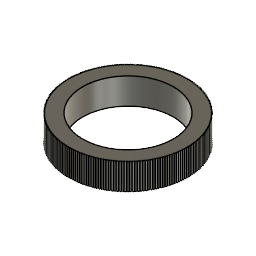
tyre (Autodesk Fusion 360 design; units mm, degrees)
Autodesk Fusion 360 part; units mm, degrees
note: some values were not read from the file. Set by a fixed rule: which sketch regions a step uses.
sketch "Sketch1" plane through (0, 0, 0) normal (0, 0, 1) x (1, 0, 0)
  circle A0 centre (0, 0) radius 17.25
  circle A1 centre (0, 0) radius 22.5
  dimension "d1" = 34.5
  dimension "d2" = 45
  constraint coincident A0.centre A1.centre
  constraint concentric A0 A1
  measures "d1" diameter of A0
  measures "d2" diameter of A1
extrude "Extrude1" add sketch "Sketch1" along normal blind 8
extrude "Extrude2" add 1 faces at (20.602, -1.9748, 8) along direction (0, 0, 1) blind 2
sketch "Sketch2" plane through (0, 0, 10) normal (0, 0, 1) x (-1, 0, 0)
  circle A0 centre (0, 0) radius 17.25
  circle A1 centre (0, 0) radius 22.5
  circle A2 centre (0, -22.5) radius 0.25
  circle A3 centre (0.7067, -22.4889) radius 0.25
  circle A4 centre (1.4128, -22.4556) radius 0.25
  circle A5 centre (2.1174, -22.4001) radius 0.25
  circle A6 centre (2.82, -22.3226) radius 0.25
  circle A7 centre (3.5198, -22.223) radius 0.25
  circle A8 centre (4.2161, -22.1015) radius 0.25
  circle A9 centre (4.9082, -21.9581) radius 0.25
  circle A10 centre (5.5955, -21.7931) radius 0.25
  circle A11 centre (6.2773, -21.6066) radius 0.25
  circle A12 centre (6.9529, -21.3988) radius 0.25
  circle A13 centre (7.6216, -21.1698) radius 0.25
  circle A14 centre (8.2828, -20.92) radius 0.25
  circle A15 centre (8.9358, -20.6495) radius 0.25
  circle A16 centre (9.58, -20.3586) radius 0.25
  circle A17 centre (10.2148, -20.0476) radius 0.25
  circle A18 centre (10.8395, -19.7169) radius 0.25
  circle A19 centre (11.4534, -19.3667) radius 0.25
  circle A20 centre (12.0561, -18.9974) radius 0.25
  circle A21 centre (12.6469, -18.6093) radius 0.25
  circle A22 centre (13.2252, -18.2029) radius 0.25
  circle A23 centre (13.7904, -17.7785) radius 0.25
  circle A24 centre (14.342, -17.3365) radius 0.25
  circle A25 centre (14.8795, -16.8775) radius 0.25
  circle A26 centre (15.4023, -16.4018) radius 0.25
  circle A27 centre (15.9099, -15.9099) radius 0.25
  circle A28 centre (16.4018, -15.4023) radius 0.25
  circle A29 centre (16.8775, -14.8795) radius 0.25
  circle A30 centre (17.3365, -14.342) radius 0.25
  circle A31 centre (17.7785, -13.7904) radius 0.25
  circle A32 centre (18.2029, -13.2252) radius 0.25
  circle A33 centre (18.6093, -12.6469) radius 0.25
  circle A34 centre (18.9974, -12.0561) radius 0.25
  circle A35 centre (19.3667, -11.4534) radius 0.25
  circle A36 centre (19.7169, -10.8395) radius 0.25
  circle A37 centre (20.0476, -10.2148) radius 0.25
  circle A38 centre (20.3586, -9.58) radius 0.25
  circle A39 centre (20.6495, -8.9358) radius 0.25
  circle A40 centre (20.92, -8.2828) radius 0.25
  circle A41 centre (21.1698, -7.6216) radius 0.25
  circle A42 centre (21.3988, -6.9529) radius 0.25
  circle A43 centre (21.6066, -6.2773) radius 0.25
  circle A44 centre (21.7931, -5.5955) radius 0.25
  circle A45 centre (21.9581, -4.9082) radius 0.25
  circle A46 centre (22.1015, -4.2161) radius 0.25
  circle A47 centre (22.223, -3.5198) radius 0.25
  circle A48 centre (22.3226, -2.82) radius 0.25
  circle A49 centre (22.4001, -2.1174) radius 0.25
  circle A50 centre (22.4556, -1.4128) radius 0.25
  circle A51 centre (22.4889, -0.7067) radius 0.25
  circle A52 centre (22.5, 0) radius 0.25
  circle A53 centre (22.4889, 0.7067) radius 0.25
  circle A54 centre (22.4556, 1.4128) radius 0.25
  circle A55 centre (22.4001, 2.1174) radius 0.25
  circle A56 centre (22.3226, 2.82) radius 0.25
  circle A57 centre (22.223, 3.5198) radius 0.25
  circle A58 centre (22.1015, 4.2161) radius 0.25
  circle A59 centre (21.9581, 4.9082) radius 0.25
  circle A60 centre (21.7931, 5.5955) radius 0.25
  circle A61 centre (21.6066, 6.2773) radius 0.25
  circle A62 centre (21.3988, 6.9529) radius 0.25
  circle A63 centre (21.1698, 7.6216) radius 0.25
  circle A64 centre (20.92, 8.2828) radius 0.25
  circle A65 centre (20.6495, 8.9358) radius 0.25
  circle A66 centre (20.3586, 9.58) radius 0.25
  circle A67 centre (20.0476, 10.2148) radius 0.25
  circle A68 centre (19.7169, 10.8395) radius 0.25
  circle A69 centre (19.3667, 11.4534) radius 0.25
  circle A70 centre (18.9974, 12.0561) radius 0.25
  circle A71 centre (18.6093, 12.6469) radius 0.25
  circle A72 centre (18.2029, 13.2252) radius 0.25
  circle A73 centre (17.7785, 13.7904) radius 0.25
  circle A74 centre (17.3365, 14.342) radius 0.25
  circle A75 centre (16.8775, 14.8795) radius 0.25
  circle A76 centre (16.4018, 15.4023) radius 0.25
  circle A77 centre (15.9099, 15.9099) radius 0.25
  circle A78 centre (15.4023, 16.4018) radius 0.25
  circle A79 centre (14.8795, 16.8775) radius 0.25
  circle A80 centre (14.342, 17.3365) radius 0.25
  circle A81 centre (13.7904, 17.7785) radius 0.25
  circle A82 centre (13.2252, 18.2029) radius 0.25
  circle A83 centre (12.6469, 18.6093) radius 0.25
  circle A84 centre (12.0561, 18.9974) radius 0.25
  circle A85 centre (11.4534, 19.3667) radius 0.25
  circle A86 centre (10.8395, 19.7169) radius 0.25
  circle A87 centre (10.2148, 20.0476) radius 0.25
  circle A88 centre (9.58, 20.3586) radius 0.25
  circle A89 centre (8.9358, 20.6495) radius 0.25
  circle A90 centre (8.2828, 20.92) radius 0.25
  circle A91 centre (7.6216, 21.1698) radius 0.25
  circle A92 centre (6.9529, 21.3988) radius 0.25
  circle A93 centre (6.2773, 21.6066) radius 0.25
  circle A94 centre (5.5955, 21.7931) radius 0.25
  circle A95 centre (4.9082, 21.9581) radius 0.25
  circle A96 centre (4.2161, 22.1015) radius 0.25
  circle A97 centre (3.5198, 22.223) radius 0.25
  circle A98 centre (2.82, 22.3226) radius 0.25
  circle A99 centre (2.1174, 22.4001) radius 0.25
  circle A100 centre (1.4128, 22.4556) radius 0.25
  circle A101 centre (0.7067, 22.4889) radius 0.25
  circle A102 centre (0, 22.5) radius 0.25
  circle A103 centre (-0.7067, 22.4889) radius 0.25
  circle A104 centre (-1.4128, 22.4556) radius 0.25
  circle A105 centre (-2.1174, 22.4001) radius 0.25
  circle A106 centre (-2.82, 22.3226) radius 0.25
  circle A107 centre (-3.5198, 22.223) radius 0.25
  circle A108 centre (-4.2161, 22.1015) radius 0.25
  circle A109 centre (-4.9082, 21.9581) radius 0.25
  circle A110 centre (-5.5955, 21.7931) radius 0.25
  circle A111 centre (-6.2773, 21.6066) radius 0.25
  circle A112 centre (-6.9529, 21.3988) radius 0.25
  circle A113 centre (-7.6216, 21.1698) radius 0.25
  circle A114 centre (-8.2828, 20.92) radius 0.25
  circle A115 centre (-8.9358, 20.6495) radius 0.25
  circle A116 centre (-9.58, 20.3586) radius 0.25
  circle A117 centre (-10.2148, 20.0476) radius 0.25
  circle A118 centre (-10.8395, 19.7169) radius 0.25
  circle A119 centre (-11.4534, 19.3667) radius 0.25
  circle A120 centre (-12.0561, 18.9974) radius 0.25
  circle A121 centre (-12.6469, 18.6093) radius 0.25
  circle A122 centre (-13.2252, 18.2029) radius 0.25
  circle A123 centre (-13.7904, 17.7785) radius 0.25
  circle A124 centre (-14.342, 17.3365) radius 0.25
  circle A125 centre (-14.8795, 16.8775) radius 0.25
  circle A126 centre (-15.4023, 16.4018) radius 0.25
  circle A127 centre (-15.9099, 15.9099) radius 0.25
  circle A128 centre (-16.4018, 15.4023) radius 0.25
  circle A129 centre (-16.8775, 14.8795) radius 0.25
  circle A130 centre (-17.3365, 14.342) radius 0.25
  circle A131 centre (-17.7785, 13.7904) radius 0.25
  circle A132 centre (-18.2029, 13.2252) radius 0.25
  circle A133 centre (-18.6093, 12.6469) radius 0.25
  circle A134 centre (-18.9974, 12.0561) radius 0.25
  circle A135 centre (-19.3667, 11.4534) radius 0.25
  circle A136 centre (-19.7169, 10.8395) radius 0.25
  circle A137 centre (-20.0476, 10.2148) radius 0.25
  circle A138 centre (-20.3586, 9.58) radius 0.25
  circle A139 centre (-20.6495, 8.9358) radius 0.25
  circle A140 centre (-20.92, 8.2828) radius 0.25
  circle A141 centre (-21.1698, 7.6216) radius 0.25
  circle A142 centre (-21.3988, 6.9529) radius 0.25
  circle A143 centre (-21.6066, 6.2773) radius 0.25
  circle A144 centre (-21.7931, 5.5955) radius 0.25
  circle A145 centre (-21.9581, 4.9082) radius 0.25
  circle A146 centre (-22.1015, 4.2161) radius 0.25
  circle A147 centre (-22.223, 3.5198) radius 0.25
  circle A148 centre (-22.3226, 2.82) radius 0.25
  circle A149 centre (-22.4001, 2.1174) radius 0.25
  circle A150 centre (-22.4556, 1.4128) radius 0.25
  circle A151 centre (-22.4889, 0.7067) radius 0.25
  circle A152 centre (-22.5, 0) radius 0.25
  circle A153 centre (-22.4889, -0.7067) radius 0.25
  circle A154 centre (-22.4556, -1.4128) radius 0.25
  circle A155 centre (-22.4001, -2.1174) radius 0.25
  circle A156 centre (-22.3226, -2.82) radius 0.25
  circle A157 centre (-22.223, -3.5198) radius 0.25
  circle A158 centre (-22.1015, -4.2161) radius 0.25
  circle A159 centre (-21.9581, -4.9082) radius 0.25
  circle A160 centre (-21.7931, -5.5955) radius 0.25
  circle A161 centre (-21.6066, -6.2773) radius 0.25
  circle A162 centre (-21.3988, -6.9529) radius 0.25
  circle A163 centre (-21.1698, -7.6216) radius 0.25
  circle A164 centre (-20.92, -8.2828) radius 0.25
  circle A165 centre (-20.6495, -8.9358) radius 0.25
  circle A166 centre (-20.3586, -9.58) radius 0.25
  circle A167 centre (-20.0476, -10.2148) radius 0.25
  circle A168 centre (-19.7169, -10.8395) radius 0.25
  circle A169 centre (-19.3667, -11.4534) radius 0.25
  circle A170 centre (-18.9974, -12.0561) radius 0.25
  circle A171 centre (-18.6093, -12.6469) radius 0.25
  circle A172 centre (-18.2029, -13.2252) radius 0.25
  circle A173 centre (-17.7785, -13.7904) radius 0.25
  circle A174 centre (-17.3365, -14.342) radius 0.25
  circle A175 centre (-16.8775, -14.8795) radius 0.25
  circle A176 centre (-16.4018, -15.4023) radius 0.25
  circle A177 centre (-15.9099, -15.9099) radius 0.25
  circle A178 centre (-15.4023, -16.4018) radius 0.25
  circle A179 centre (-14.8795, -16.8775) radius 0.25
  circle A180 centre (-14.342, -17.3365) radius 0.25
  circle A181 centre (-13.7904, -17.7785) radius 0.25
  circle A182 centre (-13.2252, -18.2029) radius 0.25
  circle A183 centre (-12.6469, -18.6093) radius 0.25
  circle A184 centre (-12.0561, -18.9974) radius 0.25
  circle A185 centre (-11.4534, -19.3667) radius 0.25
  circle A186 centre (-10.8395, -19.7169) radius 0.25
  circle A187 centre (-10.2148, -20.0476) radius 0.25
  circle A188 centre (-9.58, -20.3586) radius 0.25
  circle A189 centre (-8.9358, -20.6495) radius 0.25
  circle A190 centre (-8.2828, -20.92) radius 0.25
  circle A191 centre (-7.6216, -21.1698) radius 0.25
  circle A192 centre (-6.9529, -21.3988) radius 0.25
  circle A193 centre (-6.2773, -21.6066) radius 0.25
  circle A194 centre (-5.5955, -21.7931) radius 0.25
  circle A195 centre (-4.9082, -21.9581) radius 0.25
  circle A196 centre (-4.2161, -22.1015) radius 0.25
  circle A197 centre (-3.5198, -22.223) radius 0.25
  circle A198 centre (-2.82, -22.3226) radius 0.25
  circle A199 centre (-2.1174, -22.4001) radius 0.25
  circle A200 centre (-1.4128, -22.4556) radius 0.25
  circle A201 centre (-0.7067, -22.4889) radius 0.25
  dimension "d7" = 0.5
  dimension "d9" = 360
  constraint coincident A1 A2.centre
  measures "d7" diameter of A2
extrude "Extrude3" add sketch "Sketch2" 1 faces at (20.602, -1.9748, 10) against normal blind 10
